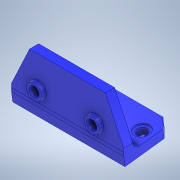
# Autodesk Inventor part: front TOF mount
Saved by Autodesk Inventor 2022.6 (Build 266554000, 554)
## iProperties
Created: 2024-11-19
Part Number: front TOF mount
Material: Generic
Document SubType Name: Modeling
Designer: Admin
Density: 1 g/cm^3
Appearance: Blue - Wall Paint - Glossy
Author: Admin
Autodesk Inventor part; units mm, degrees
ref_plane "YZ Plane" through (0, 0, 0) normal (1, 0, 0) x (0, 1, 0)
ref_plane "XZ Plane" through (0, 0, 0) normal (0, 1, 0) x (-1, 0, 0)
ref_plane "XY Plane" through (0, 0, 0) normal (0, 0, 1) x (1, 0, 0)
sketch "Sketch1" plane through (0, 0, 0) normal (1, 0, 0) x (0, 1, 0)
  line L0 (0, 0) -> (-3, 0)
  line L1 (-3, 0) -> (-3, -16)
  line L2 (-3, -16) -> (0, -16)
  line L3 (0, -16) -> (0, 0)
  line L4 (0, 0) -> (15, 0)
  line L5 (15, 0) -> (15, -3)
  line L6 (15, -3) -> (0, -3)
  line L7 (0, -3) -> (0, 0)
  point P0 (15, -1.5)
  dimension "d0" = 3
  dimension "d1" = 3
  dimension "d2" = 16
  dimension "d3" = 18
  constraints: 16 end point, 4 parallel, 2 horizontal, 2 perpendicular, 1 midpoint
  measures "d0" distance of L2.end L1.end
  measures "d1" distance of L4.end L5.end
  measures "d2" distance of L0.end L1.end
  measures "d3" distance from line of L1 point (15, -1.5)
extrude "Extrusion1" add sketch "Sketch1" along normal mid plane 37
sketch "Sketch3" plane through (-18.5, 0, -3) normal (0, 1, 0) x (1, 0, 0)
  line L0 (18.5, 16.2) -> (18.5, -6.2) projected
  line L1 (0, 0) -> (37, 0) projected
  point P0 (18.5, -3)
  point P1 (33.5, 6.5)
  point P2 (3.5, 6.5)
  dimension "d16" = 6.5
  dimension "d17" = 30
  constraints: 1 horizontal alignment, 1 symmetric about line
  measures "d16" distance from line of L1 point (33.5, 6.5)
  measures "d17" distance of point (3.5, 6.5) point (33.5, 6.5)
hole "mounting holes" at (15, 0, -9.5) at (-15, 0, -9.5) direction (0, -1, 0) diameter 3.4 end through all counterbore diameter 5 counterbore depth 0.5
sketch "Sketch4" plane through (18.5, 0, -3) normal (0, 0, -1) x (-1, 0, 0)
  line L0 (37, 0) -> (0, 0) projected
  line L1 (0, -3) -> (0, 0) projected
  line L2 (37, -3) -> (0, -3) projected
  line L3 (37, 0) -> (37, -3) projected
  line L4 (0, 15) -> (0, -3) projected
  line L5 (0, 1) -> (37, 1)
  point P0 (18.5, 0)
  point P1 (0, 4)
  dimension "d31" = 1
  constraints: 2 end point, 1 horizontal, 1 point on line
  measures "d31" distance between parallel lines of L0 L5
chamfer "Chamfer3" distance 3 angle 45 2 edges at (18.5, -1.5, -16) (-18.5, -1.5, -16)
chamfer "Chamfer4" distance 6 angle 65 2 edges at (18.5, 15, -1.5) (-18.5, 15, -1.5) measured on face at (18, 15, -1.5) measured on face at (-18, 15, -1.5)
sketch "Sketch12" plane through (-18.5, -3, 0) normal (0, 0, 1) x (1, 0, 0)
  line L0 (18.5, 21.6) -> (18.5, -3.6) projected
  line L1 (31, 3) -> (36, 3) projected
  line L2 (1, 3) -> (6, 3) projected
  line L3 (0, 3) -> (3, 3) projected
  line L4 (0, 3) -> (37, 3) projected
  line L5 (34, 3) -> (37, 3) projected
  line L6 (3, 3) -> (34, 3) projected
  point P0 (18.5, 3)
  point P1 (9, 8)
  point P2 (28, 8)
  dimension "d84" = 19
  dimension "d85" = 5
  constraints: 1 horizontal alignment, 1 symmetric about line
  measures "d84" distance of point (28, 8) point (9, 8)
  measures "d85" distance from line of L4 point (9, 8)
hole "Hole4" at (-9.5, 5, 0) at (9.5, 5, 0) direction (0, 0, -1) diameter 3.4 end through all
sketch "Sketch13" plane through (-18.5, -3, 0) normal (0, 0, 1) x (1, 0, 0)
  circle A0 centre (9, 8) radius 1.7 projected
  circle A1 centre (28, 8) radius 1.7 projected
  line L0 (0, 5.133) -> (6, 18) projected
  line L1 (0, 0) -> (0, 5.133) projected
  line L2 (0, 0) -> (37, 0) projected
  line L3 (37, 5.133) -> (37, 0) projected
  line L4 (31, 18) -> (37, 5.133) projected
  line L5 (31, 18) -> (6, 18) projected
  circle A2 centre (9, 8) radius 2.5
  circle A3 centre (28, 8) radius 2.5
  point P0 (18.5, 3)
  dimension "d93" = 5
  dimension "d94" = 5
  constraints: 2 centre point, 2 coincident
  measures "d93" diameter of A2
  measures "d94" diameter of A3
extrude "Extrusion5" add sketch "Sketch13" along normal blind 1.5 contours A2 | A3
bend part "Bend Part2" radius 7 angle 7 line through (18.5, 1, -3) along (-1, 0, 0) centre toward (0, 0, -1) moving side (0, -1, 0) both sides no
sketch "Sketch14" plane through (0, 0, 0) normal (1, 0, 0) x (0, 1, 0)
  line L0 (2.133, -3) -> (15, -3) projected
  line L1 (1.2219, -12.9953) -> (0.0032, -3.0698) projected
  line L2 (0.4907, -7.04) -> (1.1, -12.0027) projected
  line L3 (0.9769, -11) -> (12.4021, -3)
  point P0 (0, 0)
  dimension "d108" = 8
  dimension "d109" = 35
  constraints: 2 end point, 2 point on line
  measures "d108" distance from line of L0 L3.start
  measures "d109" angle of L0 L3
extrude "Rib3" add sketch "Sketch14" along normal mid plane 2 rib yes fills toward (6.6608, -6.959) open curves L3
fillet "Fillet4" radius 2 8 edges at (9.75, 0.0032, -3.0698) (-9.75, 0.0032, -3.0698) (1, 0.5727, -3.0131) (1, 0.0751, -3.061) (1, 6.701, -3) (-1, 0.5727, -3.0131) (-1, 0.0751, -3.061) (-1, 6.701, -3)
body "Solid1"
